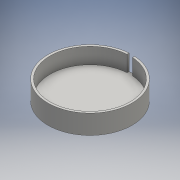
# Autodesk Inventor part: pruebaCargadorReceptor
Saved by Autodesk Inventor 2016 (Build 200138000, 138)
## iProperties
Created: 2016-04-24
Part Number: pruebaCargadorReceptor
Material: Generic
Document SubType Name: Modeling
Designer: Freddy Chang
Density: 1 g/cm^3
Appearance: Default
Author: Freddy Chang
Autodesk Inventor part; units mm, degrees
ref_plane "YZ Plane" through (0, 0, 0) normal (1, 0, 0) x (0, 1, 0)
ref_plane "XZ Plane" through (0, 0, 0) normal (0, 1, 0) x (-1, 0, 0)
ref_plane "XY Plane" through (0, 0, 0) normal (0, 0, 1) x (1, 0, 0)
sketch "Sketch1" plane through (0, 0, 0) normal (0, 0, 1) x (1, 0, 0)
  circle A0 centre (0, 0) radius 25
  dimension "d0" = 50
  constraints: 1 centre point, 1 coincident
  measures "d0" diameter of A0
extrude "Extrusion1" add sketch "Sketch1" along normal blind 11.5
sketch "Sketch2" plane through (0, 0, 11.5) normal (0, 0, 1) x (1, 0, 0)
  arc A0 (-1.6631, 23.6917) -> (1.6631, 23.6917) centre (0, 0) ccw
  line L0 (1.6631, 23.6917) -> (-1.6631, 23.6917)
  dimension "d4" = 47.5
  dimension "d8" = 23.6917
  constraints: 2 end point, 2 point on circle, 1 centre point, 1 coincident, 1 horizontal
  measures "d4" diameter of A0
  measures "d8" distance from line of point (0, 0) L0
extrude "Extrusion2" cut sketch "Sketch2" against normal blind 9.5
sketch "Sketch3" plane through (-1.6631, 23.6917, 11.5) normal (0, -1, 0) x (1, 0, 0)
  line L0 (0, 0) -> (3.3261, 0)
  line L1 (3.3261, 0) -> (3.3261, -9.5)
  line L2 (3.3261, -9.5) -> (0, -9.5)
  line L3 (0, -9.5) -> (0, 0)
  point P0 (1.6631, -11.5)
  dimension "d9" = 9.5
  dimension "d10" = 3.3261
  constraints: 8 end point, 2 parallel, 1 horizontal, 1 perpendicular
  measures "d9" distance between parallel lines of L2 L0
  measures "d10" distance between parallel lines of L1 L3
extrude "Extrusion3" cut sketch "Sketch3" against normal blind 1.5
body "Solid1"
